Autodesk Fusion 360 part; units mm, degrees
(part 3 of 3)
sketch "Boceto17" plane through (176.3664, 0, 0) normal (1, 0, 0) x (0, 0, -1)
  line L0 (-292.5, -33.6129) -> (-292.5, -30.6129)
  line L1 (-292.5, -30.6129) -> (-354.5, -30.6129)
  line L2 (-354.5, -30.6129) -> (-354.5, -33.6129)
  line L3 (-354.5, -33.6129) -> (-292.5, -33.6129)
  line L4 (-292.5, -77.1129) -> (-292.5, 0.3871)
  line L5 (-292.5, 0.3871) -> (-357.5, 0.3871)
  line L6 (-357.5, 0.3871) -> (-357.5, -77.1129)
  line L7 (-357.5, -77.1129) -> (-292.5, -77.1129)
  line L8 (-347.5, -51.3533) -> (-347.5, -60.0136)
  line L9 (-347.5, -60.0136) -> (-352.5, -62.9003)
  line L10 (-352.5, -62.9003) -> (-352.5, -48.4666)
  line L11 (-352.5, -48.4666) -> (-347.5, -51.3533)
  line L12 (-325, -64.3437) -> (-317.5, -68.6738)
  line L13 (-317.5, -68.6738) -> (-317.5, -72.1129)
  line L14 (-317.5, -72.1129) -> (-332.5, -72.1129)
  line L15 (-332.5, -72.1129) -> (-332.5, -68.6738)
  line L16 (-332.5, -68.6738) -> (-325, -64.3437)
  line L17 (-305, -64.3437) -> (-297.5, -68.6738)
  line L18 (-297.5, -68.6738) -> (-297.5, -72.1129)
  line L19 (-297.5, -72.1129) -> (-312.5, -72.1129)
  line L20 (-312.5, -72.1129) -> (-312.5, -68.6738)
  line L21 (-312.5, -68.6738) -> (-305, -64.3437)
  line L22 (-327.5, -51.3533) -> (-327.5, -60.0136)
  line L23 (-327.5, -60.0136) -> (-335, -64.3437)
  line L24 (-335, -64.3437) -> (-342.5, -60.0136)
  line L25 (-342.5, -60.0136) -> (-342.5, -51.3533)
  line L26 (-342.5, -51.3533) -> (-335, -47.0232)
  line L27 (-335, -47.0232) -> (-327.5, -51.3533)
  line L28 (-345, -64.3437) -> (-337.5, -68.6738)
  line L29 (-337.5, -68.6738) -> (-337.5, -72.1129)
  line L30 (-337.5, -72.1129) -> (-352.5, -72.1129)
  line L31 (-352.5, -72.1129) -> (-352.5, -68.6738)
  line L32 (-352.5, -68.6738) -> (-345, -64.3437)
  line L33 (-302.5, -60.0136) -> (-302.5, -51.3533)
  line L34 (-302.5, -51.3533) -> (-297.5, -48.4666)
  line L35 (-297.5, -48.4666) -> (-297.5, -62.9003)
  line L36 (-297.5, -62.9003) -> (-302.5, -60.0136)
  line L37 (-307.5, -51.3533) -> (-307.5, -60.0136)
  line L38 (-307.5, -60.0136) -> (-315, -64.3437)
  line L39 (-315, -64.3437) -> (-322.5, -60.0136)
  line L40 (-322.5, -60.0136) -> (-322.5, -51.3533)
  line L41 (-322.5, -51.3533) -> (-315, -47.0232)
  line L42 (-315, -47.0232) -> (-307.5, -51.3533)
  line L43 (-297.5, -4.6129) -> (-297.5, -8.052)
  line L44 (-297.5, -8.052) -> (-305, -12.3822)
  line L45 (-305, -12.3822) -> (-312.5, -8.052)
  line L46 (-312.5, -8.052) -> (-312.5, -4.6129)
  line L47 (-312.5, -4.6129) -> (-297.5, -4.6129)
  line L48 (-317.5, -4.6129) -> (-317.5, -8.052)
  line L49 (-317.5, -8.052) -> (-325, -12.3822)
  line L50 (-325, -12.3822) -> (-332.5, -8.052)
  line L51 (-332.5, -8.052) -> (-332.5, -4.6129)
  line L52 (-332.5, -4.6129) -> (-317.5, -4.6129)
  line L53 (-337.5, -4.6129) -> (-337.5, -8.052)
  line L54 (-337.5, -8.052) -> (-345, -12.3822)
  line L55 (-345, -12.3822) -> (-352.5, -8.052)
  line L56 (-352.5, -8.052) -> (-352.5, -4.6129)
  line L57 (-352.5, -4.6129) -> (-337.5, -4.6129)
  line L58 (-298.6195, -27.6129) -> (-302.5, -25.3725)
  line L59 (-302.5, -25.3725) -> (-302.5, -16.7123)
  line L60 (-302.5, -16.7123) -> (-297.5, -13.8255)
  line L61 (-297.5, -13.8255) -> (-297.5, -27.6129)
  line L62 (-297.5, -27.6129) -> (-298.6195, -27.6129)
  line L63 (-351.3805, -27.6129) -> (-352.5, -27.6129)
  line L64 (-352.5, -27.6129) -> (-352.5, -13.8255)
  line L65 (-352.5, -13.8255) -> (-347.5, -16.7123)
  line L66 (-347.5, -16.7123) -> (-347.5, -25.3725)
  line L67 (-347.5, -25.3725) -> (-351.3805, -27.6129)
  line L68 (-318.6195, -27.6129) -> (-322.5, -25.3725)
  line L69 (-322.5, -25.3725) -> (-322.5, -16.7123)
  line L70 (-322.5, -16.7123) -> (-315, -12.3822)
  line L71 (-315, -12.3822) -> (-307.5, -16.7123)
  line L72 (-307.5, -16.7123) -> (-307.5, -25.3725)
  line L73 (-307.5, -25.3725) -> (-311.3805, -27.6129)
  line L74 (-311.3805, -27.6129) -> (-318.6195, -27.6129)
  line L75 (-338.6195, -27.6129) -> (-342.5, -25.3725)
  line L76 (-342.5, -25.3725) -> (-342.5, -16.7123)
  line L77 (-342.5, -16.7123) -> (-335, -12.3822)
  line L78 (-335, -12.3822) -> (-327.5, -16.7123)
  line L79 (-327.5, -16.7123) -> (-327.5, -25.3725)
  line L80 (-327.5, -25.3725) -> (-331.3805, -27.6129)
  line L81 (-331.3805, -27.6129) -> (-338.6195, -27.6129)
  line L82 (-337.5, -36.6129) -> (-337.5, -42.693)
  line L83 (-337.5, -42.693) -> (-345, -47.0232)
  line L84 (-345, -47.0232) -> (-352.5, -42.693)
  line L85 (-352.5, -42.693) -> (-352.5, -36.6129)
  line L86 (-352.5, -36.6129) -> (-337.5, -36.6129)
  line L87 (-317.5, -36.6129) -> (-317.5, -42.693)
  line L88 (-317.5, -42.693) -> (-325, -47.0232)
  line L89 (-325, -47.0232) -> (-332.5, -42.693)
  line L90 (-332.5, -42.693) -> (-332.5, -36.6129)
  line L91 (-332.5, -36.6129) -> (-317.5, -36.6129)
  line L92 (-297.5, -36.6129) -> (-297.5, -42.693)
  line L93 (-297.5, -42.693) -> (-305, -47.0232)
  line L94 (-305, -47.0232) -> (-312.5, -42.693)
  line L95 (-312.5, -42.693) -> (-312.5, -36.6129)
  line L96 (-312.5, -36.6129) -> (-297.5, -36.6129)
  line L97 (-344.5, -30.6129) -> (-302.5, -30.6129)
  line L98 (-302.5, -30.6129) -> (-302.5, -33.6129)
  line L99 (-302.5, -33.6129) -> (-344.5, -33.6129)
  line L100 (-344.5, -33.6129) -> (-344.5, -30.6129)
extrude "Extruir15" add sketch "Boceto17" along normal blind 3 contours L1 L3 L97 L98 L99 L100 bodies 7
sketch "Boceto18" plane through (-0.6336, 0, 0) normal (-1, 0, 0) x (0, 0, 1)
  line L0 (337.5, -8.052) -> (337.5, -4.6129)
  line L1 (337.5, -4.6129) -> (352.5, -4.6129)
  line L2 (352.5, -4.6129) -> (352.5, -8.052)
  line L3 (352.5, -8.052) -> (345, -12.3822)
  line L4 (345, -12.3822) -> (337.5, -8.052)
  line L5 (307.5, -25.3725) -> (307.5, -16.7123)
  line L6 (307.5, -16.7123) -> (315, -12.3822)
  line L7 (315, -12.3822) -> (322.5, -16.7123)
  line L8 (322.5, -16.7123) -> (322.5, -25.3725)
  line L9 (322.5, -25.3725) -> (315, -29.7027)
  line L10 (315, -29.7027) -> (307.5, -25.3725)
  line L11 (347.5, -60.0136) -> (347.5, -51.3533)
  line L12 (347.5, -51.3533) -> (352.5, -48.4666)
  line L13 (352.5, -48.4666) -> (352.5, -62.9003)
  line L14 (352.5, -62.9003) -> (347.5, -60.0136)
  line L15 (317.5, -68.6738) -> (325, -64.3437)
  line L16 (325, -64.3437) -> (332.5, -68.6738)
  line L17 (332.5, -68.6738) -> (332.5, -72.1129)
  line L18 (332.5, -72.1129) -> (317.5, -72.1129)
  line L19 (317.5, -72.1129) -> (317.5, -68.6738)
  line L20 (297.5, -68.6738) -> (305, -64.3437)
  line L21 (305, -64.3437) -> (312.5, -68.6738)
  line L22 (312.5, -68.6738) -> (312.5, -72.1129)
  line L23 (312.5, -72.1129) -> (297.5, -72.1129)
  line L24 (297.5, -72.1129) -> (297.5, -68.6738)
  line L25 (327.5, -60.0136) -> (327.5, -51.3533)
  line L26 (327.5, -51.3533) -> (335, -47.0232)
  line L27 (335, -47.0232) -> (342.5, -51.3533)
  line L28 (342.5, -51.3533) -> (342.5, -60.0136)
  line L29 (342.5, -60.0136) -> (335, -64.3437)
  line L30 (335, -64.3437) -> (327.5, -60.0136)
  line L31 (337.5, -42.693) -> (337.5, -34.0328)
  line L32 (337.5, -34.0328) -> (345, -29.7027)
  line L33 (345, -29.7027) -> (352.5, -34.0328)
  line L34 (352.5, -34.0328) -> (352.5, -42.693)
  line L35 (352.5, -42.693) -> (345, -47.0232)
  line L36 (345, -47.0232) -> (337.5, -42.693)
  line L37 (347.5, -25.3725) -> (347.5, -16.7123)
  line L38 (347.5, -16.7123) -> (352.5, -13.8255)
  line L39 (352.5, -13.8255) -> (352.5, -28.2593)
  line L40 (352.5, -28.2593) -> (347.5, -25.3725)
  line L41 (317.5, -8.052) -> (317.5, -4.6129)
  line L42 (317.5, -4.6129) -> (332.5, -4.6129)
  line L43 (332.5, -4.6129) -> (332.5, -8.052)
  line L44 (332.5, -8.052) -> (325, -12.3822)
  line L45 (325, -12.3822) -> (317.5, -8.052)
  line L46 (297.5, -28.2593) -> (297.5, -13.8255)
  line L47 (297.5, -13.8255) -> (302.5, -16.7123)
  line L48 (302.5, -16.7123) -> (302.5, -25.3725)
  line L49 (302.5, -25.3725) -> (297.5, -28.2593)
  line L50 (297.5, -42.693) -> (297.5, -34.0328)
  line L51 (297.5, -34.0328) -> (305, -29.7027)
  line L52 (305, -29.7027) -> (312.5, -34.0328)
  line L53 (312.5, -34.0328) -> (312.5, -42.693)
  line L54 (312.5, -42.693) -> (305, -47.0232)
  line L55 (305, -47.0232) -> (297.5, -42.693)
  line L56 (337.5, -68.6738) -> (345, -64.3437)
  line L57 (345, -64.3437) -> (352.5, -68.6738)
  line L58 (352.5, -68.6738) -> (352.5, -72.1129)
  line L59 (352.5, -72.1129) -> (337.5, -72.1129)
  line L60 (337.5, -72.1129) -> (337.5, -68.6738)
  line L61 (302.5, -51.3533) -> (302.5, -60.0136)
  line L62 (302.5, -60.0136) -> (297.5, -62.9003)
  line L63 (297.5, -62.9003) -> (297.5, -48.4666)
  line L64 (297.5, -48.4666) -> (302.5, -51.3533)
  line L65 (307.5, -60.0136) -> (307.5, -51.3533)
  line L66 (307.5, -51.3533) -> (315, -47.0232)
  line L67 (315, -47.0232) -> (322.5, -51.3533)
  line L68 (322.5, -51.3533) -> (322.5, -60.0136)
  line L69 (322.5, -60.0136) -> (315, -64.3437)
  line L70 (315, -64.3437) -> (307.5, -60.0136)
  line L71 (332.5, -42.693) -> (325, -47.0232)
  line L72 (325, -47.0232) -> (317.5, -42.693)
  line L73 (317.5, -42.693) -> (317.5, -34.0328)
  line L74 (317.5, -34.0328) -> (325, -29.7027)
  line L75 (325, -29.7027) -> (332.5, -34.0328)
  line L76 (332.5, -34.0328) -> (332.5, -42.693)
  line L77 (327.5, -25.3725) -> (327.5, -16.7123)
  line L78 (327.5, -16.7123) -> (335, -12.3822)
  line L79 (335, -12.3822) -> (342.5, -16.7123)
  line L80 (342.5, -16.7123) -> (342.5, -25.3725)
  line L81 (342.5, -25.3725) -> (335, -29.7027)
  line L82 (335, -29.7027) -> (327.5, -25.3725)
  line L83 (297.5, -8.052) -> (297.5, -4.6129)
  line L84 (297.5, -4.6129) -> (312.5, -4.6129)
  line L85 (312.5, -4.6129) -> (312.5, -8.052)
  line L86 (312.5, -8.052) -> (305, -12.3822)
  line L87 (305, -12.3822) -> (297.5, -8.052)
  line L88 (357.5, 0.3871) -> (292.5, 0.3871)
  line L89 (292.5, 0.3871) -> (292.5, -77.1129)
  line L90 (292.5, -77.1129) -> (357.5, -77.1129)
  line L91 (357.5, -77.1129) -> (357.5, 0.3871)
  line L92 (292.5, -77.1129) -> (292.5, 0.3871)
  line L93 (292.5, 0.3871) -> (357.5, 0.3871)
  line L94 (357.5, 0.3871) -> (357.5, -77.1129)
  line L95 (357.5, -77.1129) -> (292.5, -77.1129)
  line L96 (347.5, -51.3533) -> (347.5, -60.0136)
  line L97 (347.5, -60.0136) -> (352.5, -62.9003)
  line L98 (352.5, -62.9003) -> (352.5, -48.4666)
  line L99 (352.5, -48.4666) -> (347.5, -51.3533)
  line L100 (325, -64.3437) -> (317.5, -68.6738)
  line L101 (317.5, -68.6738) -> (317.5, -72.1129)
  line L102 (317.5, -72.1129) -> (332.5, -72.1129)
  line L103 (332.5, -72.1129) -> (332.5, -68.6738)
  line L104 (332.5, -68.6738) -> (325, -64.3437)
  line L105 (305, -64.3437) -> (297.5, -68.6738)
  line L106 (297.5, -68.6738) -> (297.5, -72.1129)
  line L107 (297.5, -72.1129) -> (312.5, -72.1129)
  line L108 (312.5, -72.1129) -> (312.5, -68.6738)
  line L109 (312.5, -68.6738) -> (305, -64.3437)
  line L110 (327.5, -51.3533) -> (327.5, -60.0136)
  line L111 (327.5, -60.0136) -> (335, -64.3437)
  line L112 (335, -64.3437) -> (342.5, -60.0136)
  line L113 (342.5, -60.0136) -> (342.5, -51.3533)
  line L114 (342.5, -51.3533) -> (335, -47.0232)
  line L115 (335, -47.0232) -> (327.5, -51.3533)
  line L116 (345, -64.3437) -> (337.5, -68.6738)
  line L117 (337.5, -68.6738) -> (337.5, -72.1129)
  line L118 (337.5, -72.1129) -> (352.5, -72.1129)
  line L119 (352.5, -72.1129) -> (352.5, -68.6738)
  line L120 (352.5, -68.6738) -> (345, -64.3437)
  line L121 (302.5, -60.0136) -> (302.5, -51.3533)
  line L122 (302.5, -51.3533) -> (297.5, -48.4666)
  line L123 (297.5, -48.4666) -> (297.5, -62.9003)
  line L124 (297.5, -62.9003) -> (302.5, -60.0136)
  line L125 (307.5, -51.3533) -> (307.5, -60.0136)
  line L126 (307.5, -60.0136) -> (315, -64.3437)
  line L127 (315, -64.3437) -> (322.5, -60.0136)
  line L128 (322.5, -60.0136) -> (322.5, -51.3533)
  line L129 (322.5, -51.3533) -> (315, -47.0232)
  line L130 (315, -47.0232) -> (307.5, -51.3533)
  line L131 (297.5, -4.6129) -> (297.5, -8.052)
  line L132 (297.5, -8.052) -> (305, -12.3822)
  line L133 (305, -12.3822) -> (312.5, -8.052)
  line L134 (312.5, -8.052) -> (312.5, -4.6129)
  line L135 (312.5, -4.6129) -> (297.5, -4.6129)
  line L136 (317.5, -4.6129) -> (317.5, -8.052)
  line L137 (317.5, -8.052) -> (325, -12.3822)
  line L138 (325, -12.3822) -> (332.5, -8.052)
  line L139 (332.5, -8.052) -> (332.5, -4.6129)
  line L140 (332.5, -4.6129) -> (317.5, -4.6129)
  line L141 (337.5, -4.6129) -> (337.5, -8.052)
  line L142 (337.5, -8.052) -> (345, -12.3822)
  line L143 (345, -12.3822) -> (352.5, -8.052)
  line L144 (352.5, -8.052) -> (352.5, -4.6129)
  line L145 (352.5, -4.6129) -> (337.5, -4.6129)
  line L146 (298.6195, -27.6129) -> (302.5, -25.3725)
  line L147 (302.5, -25.3725) -> (302.5, -16.7123)
  line L148 (302.5, -16.7123) -> (297.5, -13.8255)
  line L149 (297.5, -13.8255) -> (297.5, -27.6129)
  line L150 (297.5, -27.6129) -> (298.6195, -27.6129)
  line L151 (351.3805, -27.6129) -> (352.5, -27.6129)
  line L152 (352.5, -27.6129) -> (352.5, -13.8255)
  line L153 (352.5, -13.8255) -> (347.5, -16.7123)
  line L154 (347.5, -16.7123) -> (347.5, -25.3725)
  line L155 (347.5, -25.3725) -> (351.3805, -27.6129)
  line L156 (318.6195, -27.6129) -> (322.5, -25.3725)
  line L157 (322.5, -25.3725) -> (322.5, -16.7123)
  line L158 (322.5, -16.7123) -> (315, -12.3822)
  line L159 (315, -12.3822) -> (307.5, -16.7123)
  line L160 (307.5, -16.7123) -> (307.5, -25.3725)
  line L161 (307.5, -25.3725) -> (311.3805, -27.6129)
  line L162 (311.3805, -27.6129) -> (318.6195, -27.6129)
  line L163 (338.6195, -27.6129) -> (342.5, -25.3725)
  line L164 (342.5, -25.3725) -> (342.5, -16.7123)
  line L165 (342.5, -16.7123) -> (335, -12.3822)
  line L166 (335, -12.3822) -> (327.5, -16.7123)
  line L167 (327.5, -16.7123) -> (327.5, -25.3725)
  line L168 (327.5, -25.3725) -> (331.3805, -27.6129)
  line L169 (331.3805, -27.6129) -> (338.6195, -27.6129)
  line L170 (337.5, -36.6129) -> (337.5, -42.693)
  line L171 (337.5, -42.693) -> (345, -47.0232)
  line L172 (345, -47.0232) -> (352.5, -42.693)
  line L173 (352.5, -42.693) -> (352.5, -36.6129)
  line L174 (352.5, -36.6129) -> (337.5, -36.6129)
  line L175 (317.5, -36.6129) -> (317.5, -42.693)
  line L176 (317.5, -42.693) -> (325, -47.0232)
  line L177 (325, -47.0232) -> (332.5, -42.693)
  line L178 (332.5, -42.693) -> (332.5, -36.6129)
  line L179 (332.5, -36.6129) -> (317.5, -36.6129)
  line L180 (297.5, -36.6129) -> (297.5, -42.693)
  line L181 (297.5, -42.693) -> (305, -47.0232)
  line L182 (305, -47.0232) -> (312.5, -42.693)
  line L183 (312.5, -42.693) -> (312.5, -36.6129)
  line L184 (312.5, -36.6129) -> (297.5, -36.6129)
  line L185 (344.5, -30.6129) -> (302.5, -30.6129)
  line L186 (302.5, -30.6129) -> (302.5, -33.6129)
  line L187 (302.5, -33.6129) -> (344.5, -33.6129)
  line L188 (344.5, -33.6129) -> (344.5, -30.6129)
  line L189 (344.5, -33.6129) -> (302.5, -33.6129)
  line L190 (302.5, -33.6129) -> (302.5, -30.6129)
  line L191 (302.5, -30.6129) -> (344.5, -30.6129)
  line L192 (344.5, -30.6129) -> (344.5, -33.6129)
  line L193 (344.5, -33.6129) -> (344.5, -30.6129)
  line L194 (344.5, -33.6129) -> (302.5, -33.6129)
  line L195 (302.5, -33.6129) -> (302.5, -30.6129)
  line L196 (302.5, -30.6129) -> (344.5, -30.6129)
  line L197 (344.5, -30.6129) -> (344.5, -33.6129)
  line L198 (352.5, -36.6129) -> (357.5, -36.6129)
  line L199 (357.5, -36.6129) -> (292.5, -36.6129)
  line L200 (292.5, -36.6129) -> (292.5, -27.6129)
  line L201 (292.5, -27.6129) -> (357.5, -27.6129)
  line L202 (357.5, -27.6129) -> (357.5, -36.6129)
  constraint coincident L187.end L188.start
  constraint coincident L185.start L188.end
  constraint horizontal L194
  constraint vertical L195
  constraint horizontal L196
  constraint vertical L197
  constraint coincident L185.end L186.start
  constraint coincident L173.end L174.start
  constraint coincident L94 L198.end
  constraint perpendicular L94 L198
  constraint horizontal L199
  constraint vertical L200
  constraint horizontal L201
  constraint vertical L202
  constraint coincident L92 L200.end
extrude "Extruir16" add sketch "Boceto18" against normal blind 3 contours L9 L10 L162 L201 | L9 L10 L32 L33 L34 L39 L40 L46 L49 L50 L51 L52 L74 L75 L81 L82 L89 L91 L92 L94 L185 L186 L190 L191 L195 L196 L198 L199 L200 L201 L202 | L46 L49 L150 L201 | L81 L82 L169 L201 | L50 L51 L52 L53 L184 L186 L187 L189 L190 L194 L195 L199 | L52 L53 L73 L74 L187 L189 L194 L199 | L73 L74 L75 L76 L179 L187 L189 L194 L199 | L31 L32 L33 L34 L174 L185 L187 L188 L189 L191 L192 L193 L194 L196 L197 L199 | L51 L52 L185 L191 L196 | L31 L32 L75 L76 L187 L189 L194 L199 | L74 L75 L185 L191 L196 bodies 3
extrude "Extruir17" cut sketch "Boceto18" against normal blind 3 contours L51 L185 L186 L190 L191 L195 L196 | L51 L52 L185 L186 L187 L189 L190 L191 L194 L195 L196 | L52 L74 L185 L187 L189 L191 L194 L196 | L74 L75 L185 L187 L189 L191 L194 L196 | L32 L75 L185 L187 L189 L191 L194 L196 | L32 L185 L187 L188 L189 L191 L192 L193 L194 L196 L197 bodies 3
sketch "Boceto19" plane through (-0.6336, 0, 0) normal (-1, 0, 0) x (0, 0, 1)
  line L0 (344.5, -33.6129) -> (302.5, -33.6129)
  line L1 (302.5, -33.6129) -> (302.5, -30.6129)
  line L2 (302.5, -30.6129) -> (344.5, -30.6129)
  line L3 (344.5, -30.6129) -> (344.5, -33.6129)
extrude "Extruir18" add sketch "Boceto19" against normal blind 3 bodies 7
sketch "Boceto20" plane through (0, -33.6129, 0) normal (0, -1, 0) x (1, 0, 0)
  line L0 (136.8664, 296.5) -> (41.8664, 296.5)
  line L1 (41.8664, 296.5) -> (41.8664, 300.5)
  line L2 (41.8664, 300.5) -> (136.8664, 300.5)
  line L3 (136.8664, 300.5) -> (136.8664, 296.5)
  line L4 (2.3664, 292.5) -> (176.3664, 292.5)
  line L5 (176.3664, 354.5) -> (2.3664, 354.5)
  line L6 (7.3664, 349.5) -> (171.3664, 349.5)
  line L7 (171.3664, 349.5) -> (171.3664, 297.5)
  line L8 (7.3664, 297.5) -> (7.3664, 349.5)
  line L9 (41.8664, 296.5) -> (41.8664, 297.5)
  line L10 (141.8664, 305.5) -> (141.8664, 297.5)
  line L11 (171.3664, 297.5) -> (141.8664, 297.5)
  line L12 (36.8664, 297.5) -> (7.3664, 297.5)
  line L13 (36.8664, 297.5) -> (36.8664, 305.5)
  line L14 (7.3664, 323.5) -> (171.3664, 323.5) construction
  line L15 (80.7061, 323.5) -> (85.0363, 316)
  line L16 (85.0363, 316) -> (93.6965, 316)
  line L17 (93.6965, 316) -> (98.0267, 323.5)
  line L18 (98.0267, 323.5) -> (93.6965, 331)
  line L19 (93.6965, 331) -> (85.0363, 331)
  line L20 (85.0363, 331) -> (80.7061, 323.5)
  line L21 (89.3664, 323.5) -> (89.3664, 316) construction
  line L22 (89.3664, 323.5) -> (82.8712, 319.75) construction
  line L23 (169.6181, 349.5) -> (171.6388, 346)
  line L24 (171.6388, 341) -> (167.3087, 333.5)
  line L25 (167.3087, 333.5) -> (171.6388, 326)
  line L26 (171.6388, 321) -> (167.3087, 313.5)
  line L27 (167.3087, 313.5) -> (171.6388, 306)
  line L28 (171.6388, 301) -> (169.6181, 297.5)
  line L29 (153.4523, 349.5) -> (149.9882, 343.5)
  line L30 (149.9882, 343.5) -> (154.3183, 336)
  line L31 (154.3183, 336) -> (162.9786, 336)
  line L32 (167.3087, 343.5) -> (163.8446, 349.5)
  line L33 (162.9786, 336) -> (167.3087, 343.5)
  line L34 (162.9786, 331) -> (154.3183, 331)
  line L35 (154.3183, 331) -> (149.9882, 323.5)
  line L36 (149.9882, 323.5) -> (154.3183, 316)
  line L37 (154.3183, 316) -> (162.9786, 316)
  line L38 (167.3087, 323.5) -> (162.9786, 331)
  line L39 (162.9786, 316) -> (167.3087, 323.5)
  line L40 (162.9786, 311) -> (154.3183, 311)
  line L41 (154.3183, 311) -> (149.9882, 303.5)
  line L42 (149.9882, 303.5) -> (153.4523, 297.5)
  line L43 (167.3087, 303.5) -> (162.9786, 311)
  line L44 (163.8446, 297.5) -> (167.3087, 303.5)
  line L45 (134.9771, 349.5) -> (136.9978, 346)
  line L46 (136.9978, 346) -> (145.6581, 346)
  line L47 (145.6581, 346) -> (147.6788, 349.5)
  line L48 (145.6581, 341) -> (136.9978, 341)
  line L49 (136.9978, 341) -> (132.6677, 333.5)
  line L50 (132.6677, 333.5) -> (136.9978, 326)
  line L51 (136.9978, 326) -> (145.6581, 326)
  line L52 (149.9882, 333.5) -> (145.6581, 341)
  line L53 (145.6581, 326) -> (149.9882, 333.5)
  line L54 (145.6581, 321) -> (136.9978, 321)
  line L55 (136.9978, 321) -> (132.6677, 313.5)
  line L56 (132.6677, 313.5) -> (136.9978, 306)
  line L57 (136.9978, 306) -> (145.6581, 306)
  line L58 (149.9882, 313.5) -> (145.6581, 321)
  line L59 (145.6581, 306) -> (149.9882, 313.5)
  line L60 (145.6581, 301) -> (141.8664, 301)
  line L61 (136.9978, 301) -> (136.7091, 300.5)
  line L62 (147.6788, 297.5) -> (145.6581, 301)
  line L63 (118.8113, 349.5) -> (115.3472, 343.5)
  line L64 (115.3472, 343.5) -> (119.6773, 336)
  line L65 (119.6773, 336) -> (128.3375, 336)
  line L66 (132.6677, 343.5) -> (129.2036, 349.5)
  line L67 (128.3375, 336) -> (132.6677, 343.5)
  line L68 (128.3375, 331) -> (119.6773, 331)
  line L69 (119.6773, 331) -> (115.3472, 323.5)
  line L70 (115.3472, 323.5) -> (119.6773, 316)
  line L71 (119.6773, 316) -> (128.3375, 316)
  line L72 (132.6677, 323.5) -> (128.3375, 331)
  line L73 (128.3375, 316) -> (132.6677, 323.5)
  line L74 (128.3375, 311) -> (119.6773, 311)
  line L75 (119.6773, 311) -> (116.5019, 305.5)
  line L76 (131.513, 305.5) -> (128.3375, 311)
  line L77 (100.3361, 349.5) -> (102.3568, 346)
  line L78 (102.3568, 346) -> (111.017, 346)
  line L79 (111.017, 346) -> (113.0378, 349.5)
  line L80 (111.017, 341) -> (102.3568, 341)
  line L81 (102.3568, 341) -> (98.0267, 333.5)
  line L82 (98.0267, 333.5) -> (102.3568, 326)
  line L83 (102.3568, 326) -> (111.017, 326)
  line L84 (115.3472, 333.5) -> (111.017, 341)
  line L85 (111.017, 326) -> (115.3472, 333.5)
  line L86 (111.017, 321) -> (102.3568, 321)
  line L87 (102.3568, 321) -> (98.0267, 313.5)
  line L88 (98.0267, 313.5) -> (102.3568, 306)
  line L89 (102.3568, 306) -> (111.017, 306)
  line L90 (115.3472, 313.5) -> (111.017, 321)
  line L91 (111.017, 306) -> (115.3472, 313.5)
  line L92 (84.1703, 349.5) -> (80.7061, 343.5)
  line L93 (80.7061, 343.5) -> (85.0363, 336)
  line L94 (85.0363, 336) -> (93.6965, 336)
  line L95 (98.0267, 343.5) -> (94.5626, 349.5)
  line L96 (93.6965, 336) -> (98.0267, 343.5)
  line L97 (93.6965, 311) -> (85.0363, 311)
  line L98 (85.0363, 311) -> (81.8609, 305.5)
  line L99 (96.872, 305.5) -> (93.6965, 311)
  line L100 (65.695, 349.5) -> (67.7158, 346)
  line L101 (67.7158, 346) -> (76.376, 346)
  line L102 (76.376, 346) -> (78.3967, 349.5)
  line L103 (76.376, 341) -> (67.7158, 341)
  line L104 (67.7158, 341) -> (63.3856, 333.5)
  line L105 (63.3856, 333.5) -> (67.7158, 326)
  line L106 (67.7158, 326) -> (76.376, 326)
  line L107 (80.7061, 333.5) -> (76.376, 341)
  line L108 (76.376, 326) -> (80.7061, 333.5)
  line L109 (76.376, 321) -> (67.7158, 321)
  line L110 (67.7158, 321) -> (63.3856, 313.5)
  line L111 (63.3856, 313.5) -> (67.7158, 306)
  line L112 (67.7158, 306) -> (76.376, 306)
  line L113 (80.7061, 313.5) -> (76.376, 321)
  line L114 (76.376, 306) -> (80.7061, 313.5)
  line L115 (49.5292, 349.5) -> (46.0651, 343.5)
  line L116 (46.0651, 343.5) -> (50.3953, 336)
  line L117 (50.3953, 336) -> (59.0555, 336)
  line L118 (63.3856, 343.5) -> (59.9215, 349.5)
  line L119 (59.0555, 336) -> (63.3856, 343.5)
  line L120 (59.0555, 331) -> (50.3953, 331)
  line L121 (50.3953, 331) -> (46.0651, 323.5)
  line L122 (46.0651, 323.5) -> (50.3953, 316)
  line L123 (50.3953, 316) -> (59.0555, 316)
  line L124 (63.3856, 323.5) -> (59.0555, 331)
  line L125 (59.0555, 316) -> (63.3856, 323.5)
  line L126 (59.0555, 311) -> (50.3953, 311)
  line L127 (50.3953, 311) -> (47.2198, 305.5)
  line L128 (50.1066, 296.5) -> (50.3953, 296)
  line L129 (62.2309, 305.5) -> (59.0555, 311)
  line L130 (31.054, 349.5) -> (33.0748, 346)
  line L131 (33.0748, 346) -> (41.735, 346)
  line L132 (41.735, 346) -> (43.7557, 349.5)
  line L133 (41.735, 341) -> (33.0748, 341)
  line L134 (33.0748, 341) -> (28.7446, 333.5)
  line L135 (28.7446, 333.5) -> (33.0748, 326)
  line L136 (33.0748, 326) -> (41.735, 326)
  line L137 (46.0651, 333.5) -> (41.735, 341)
  line L138 (41.735, 326) -> (46.0651, 333.5)
  line L139 (41.735, 321) -> (33.0748, 321)
  line L140 (33.0748, 321) -> (28.7446, 313.5)
  line L141 (28.7446, 313.5) -> (33.0748, 306)
  line L142 (33.0748, 306) -> (41.735, 306)
  line L143 (46.0651, 313.5) -> (41.735, 321)
  line L144 (41.735, 306) -> (46.0651, 313.5)
  line L145 (36.8664, 301) -> (33.0748, 301)
  line L146 (33.0748, 301) -> (31.054, 297.5)
  line L147 (42.0237, 300.5) -> (41.735, 301)
  line L148 (14.8882, 349.5) -> (11.4241, 343.5)
  line L149 (11.4241, 343.5) -> (15.7542, 336)
  line L150 (15.7542, 336) -> (24.4145, 336)
  line L151 (28.7446, 343.5) -> (25.2805, 349.5)
  line L152 (24.4145, 336) -> (28.7446, 343.5)
  line L153 (24.4145, 331) -> (15.7542, 331)
  line L154 (15.7542, 331) -> (11.4241, 323.5)
  line L155 (11.4241, 323.5) -> (15.7542, 316)
  line L156 (15.7542, 316) -> (24.4145, 316)
  line L157 (28.7446, 323.5) -> (24.4145, 331)
  line L158 (24.4145, 316) -> (28.7446, 323.5)
  line L159 (24.4145, 311) -> (15.7542, 311)
  line L160 (15.7542, 311) -> (11.4241, 303.5)
  line L161 (11.4241, 303.5) -> (14.8882, 297.5)
  line L162 (28.7446, 303.5) -> (24.4145, 311)
  line L163 (25.2805, 297.5) -> (28.7446, 303.5)
  line L164 (7.094, 346) -> (9.1147, 349.5)
  line L165 (11.4241, 333.5) -> (7.094, 341)
  line L166 (7.094, 326) -> (11.4241, 333.5)
  line L167 (11.4241, 313.5) -> (7.094, 321)
  line L168 (7.094, 306) -> (11.4241, 313.5)
  line L169 (9.1147, 297.5) -> (7.094, 301)
  line L170 (59.0555, 296) -> (59.3442, 296.5)
  line L171 (36.8664, 305.5) -> (62.2309, 305.5)
  line L172 (81.8609, 305.5) -> (141.8664, 305.5)
  line L173 (81.8609, 305.5) -> (62.2309, 305.5)
  point P0 (89.3664, 323.5)
  dimension "d102" = 15
  constraint vertical L9
  constraint collinear L11 L12
  constraint coincident L1 L9.end
  constraint horizontal L14
  constraint coincident L7 L14.end
  constraint midpoint L14 P0
  constraint parallel L6 L19
  constraint coincident P0 L21.start
  constraint midpoint L16 L21.end
  constraint midpoint L15 L22.end
  constraint coincident L6 L23.start
  constraint coincident L6 L32.end
  constraint coincident L6 L29.start
  constraint coincident L6 L47.end
  constraint coincident L6 L45.start
  constraint coincident L6 L79.end
  constraint coincident L6 L77.start
  constraint coincident L6 L66.end
  constraint coincident L6 L63.start
  constraint coincident L6 L95.end
  constraint coincident L6 L92.start
  constraint coincident L6 L102.end
  constraint coincident L6 L100.start
  constraint coincident L6 L132.end
  constraint coincident L6 L118.end
  constraint coincident L6 L115.start
  constraint coincident L6 L130.start
  constraint coincident L6 L164.end
  constraint coincident L6 L151.end
  constraint coincident L6 L148.start
  constraint coincident L12 L169.start
  constraint coincident L12 L163.start
  constraint coincident L12 L161.end
  constraint coincident L12 L146.end
  constraint coincident L0 L170.end
  constraint coincident L0 L128.start
  constraint coincident L2 L147.start
  constraint coincident L13 L145.start
  constraint coincident L127.end L171
  constraint collinear L171 L172
  constraint coincident L172 L99.start
  constraint coincident L172 L76.start
  constraint coincident L172 L75.end
  constraint coincident L10 L60.end
  constraint coincident L2 L61.end
  constraint coincident L11 L62.start
  constraint coincident L11 L44.start
  constraint coincident L11 L42.end
  constraint coincident L11 L28.end
  constraint parallel L171 L173
  measures "d102" distance of L16 L19
extrude "Extruir19" cut sketch "Boceto20" against normal blind 40 contours L6 L148 L149 L150 L151 L152 | L6 L130 L131 L132 | L6 L115 L116 L117 L118 L119 | L6 L100 L101 L102 | L12 L159 L160 L161 L162 L163 | L6 L92 L93 L94 L95 L96 | L6 L77 L78 L79 | L6 L63 L64 L65 L66 L67 | L126 L127 L129 L171 | L6 L45 L46 L47 | L97 L98 L99 L172 | L6 L29 L30 L31 L32 L33 | L74 L75 L76 L172 | L11 L40 L41 L42 L43 L44 | L15 L16 L17 L18 L19 L20 | L34 L35 L36 L37 L38 L39 | L48 L49 L50 L51 L52 L53 | L54 L55 L56 L57 L58 L59 | L68 L69 L70 L71 L72 L73 | L80 L81 L82 L83 L84 L85 | L86 L87 L88 L89 L90 L91 | L103 L104 L105 L106 L107 L108 | L109 L110 L111 L112 L113 L114 | L120 L121 L122 L123 L124 L125 | L133 L134 L135 L136 L137 L138 | L139 L140 L141 L142 L143 L144 | L153 L154 L155 L156 L157 L158 bodies 7
move_face "CarasDesfase1" offset -0.15 2 faces at (136.8664, -117.6129, 314.1667) (41.8664, -117.6129, 314.1667) on bodies 6
move_face "CarasDesfase2" offset -0.15 4 faces at (178.3664, -33.6129, 316.5) (178.3664, -32.6129, 302.5) (178.3664, -30.6129, 316.5) (178.3664, -32.6129, 344.5) on bodies 2
sketch "Boceto21" plane through (0, 0, 292.5) normal (0, 0, -1) x (-1, 0, 0)
  line L0 (-42.0164, -116.6129) -> (-136.7164, -116.6129)
  line L1 (-136.7164, -116.6129) -> (-136.7164, -119.6129)
  line L2 (-136.7164, -119.6129) -> (-42.0164, -119.6129)
  line L3 (-42.0164, -119.6129) -> (-42.0164, -116.6129)
  line L4 (-89.3664, -116.6129) -> (-101.1964, -116.6129)
  line L5 (-101.1964, -116.6129) -> (-101.1964, -76.4129)
  line L6 (-101.1964, -76.4129) -> (-77.5364, -76.4129)
  line L7 (-77.5364, -76.4129) -> (-77.5364, -116.6129)
  line L8 (-77.5364, -116.6129) -> (-89.3664, -116.6129)
  dimension "d111" = 11.83
  dimension "d112" = 40.2
  dimension "d113" = 23.66
  constraint midpoint L0 L4.start
  constraint parallel L0 L4
  constraint perpendicular L0 L5
  constraint perpendicular L5 L6
  constraint coincident L0 L7.end
  constraint perpendicular L0 L7
  measures "d111" distance of L4.start L4.end
  measures "d112" distance of L4.end L5.end
  measures "d113" distance of L5.end L6.end
extrude "Extruir20" add sketch "Boceto21" against normal blind 2 contours L0 L4 L5 L6 L7 L8 bodies 6
sketch "Boceto22" plane through (0, 0, 294.5) normal (0, 0, 1) x (1, 0, 0)
  line L0 (77.5364, -76.4129) -> (77.5364, -116.6129)
  line L1 (77.5364, -116.6129) -> (101.1964, -116.6129)
  line L2 (101.1964, -116.6129) -> (101.1964, -76.4129)
  line L3 (101.1964, -76.4129) -> (77.5364, -76.4129)
  line L4 (77.5364, -76.4129) -> (82.0364, -76.4129)
  line L5 (82.0364, -76.4129) -> (82.0364, -86.4129)
  line L6 (82.0364, -86.4129) -> (77.5364, -86.4129)
  line L7 (77.5364, -86.4129) -> (77.5364, -76.4129)
  line L8 (101.1964, -76.4129) -> (96.6964, -76.4129)
  line L9 (96.6964, -76.4129) -> (96.6964, -86.4129)
  line L10 (96.6964, -86.4129) -> (101.1964, -86.4129)
  line L11 (101.1964, -86.4129) -> (101.1964, -76.4129)
  dimension "d116" = 4.5
  dimension "d117" = 10
  dimension "d118" = 4.5
  dimension "d119" = 10
  constraint horizontal L4
  constraint vertical L5
  constraint horizontal L6
  constraint vertical L7
  constraint coincident L0.start L3.end
  constraint horizontal L8
  constraint vertical L9
  constraint horizontal L10
  constraint vertical L11
  constraint coincident L2.end L3.start
  measures "d116" distance of L0.start L4.end
  measures "d117" distance of L0.start L6.end
  measures "d118" distance of L2.end L8.end
  measures "d119" distance of L2.end L10.end
extrude "Extruir21" add sketch "Boceto22" along normal blind 4.5 contours L0 L3 L4 L5 L6 L7 | L2 L3 L8 L9 L10 L11 bodies 6
sketch "Boceto23" plane through (0, -76.4129, 0) normal (0, 1, 0) x (-1, 0, 0)
  line L0 (-101.1964, 292.5) -> (-77.5364, 292.5)
  line L1 (-77.5364, 292.5) -> (-77.5364, 299)
  line L2 (-77.5364, 299) -> (-82.0364, 299)
  line L3 (-82.0364, 299) -> (-82.0364, 294.5)
  line L4 (-82.0364, 294.5) -> (-96.6964, 294.5)
  line L5 (-96.6964, 294.5) -> (-96.6964, 299)
  line L6 (-96.6964, 299) -> (-101.1964, 299)
  line L7 (-101.1964, 299) -> (-101.1964, 292.5)
  line L8 (-96.6964, 294.5) -> (-99.6964, 294.5)
  line L9 (-99.6964, 294.5) -> (-99.6964, 297.5)
  line L10 (-99.6964, 297.5) -> (-96.6964, 297.5)
  line L11 (-96.6964, 297.5) -> (-96.6964, 294.5)
  line L12 (-82.0364, 294.5) -> (-79.0364, 294.5)
  line L13 (-79.0364, 294.5) -> (-79.0364, 297.5)
  line L14 (-79.0364, 297.5) -> (-82.0364, 297.5)
  line L15 (-82.0364, 297.5) -> (-82.0364, 294.5)
  dimension "d122" = 3
  dimension "d123" = 3
  dimension "d124" = 3
  dimension "d125" = 3
  constraint horizontal L8
  constraint vertical L9
  constraint horizontal L10
  constraint vertical L11
  constraint coincident L4.end L5.start
  constraint horizontal L12
  constraint vertical L13
  constraint horizontal L14
  constraint vertical L15
  constraint coincident L3.end L4.start
  measures "d122" distance of L4.end L8.end
  measures "d123" distance of L4.end L10.end
  measures "d124" distance of L3.end L12.end
  measures "d125" distance of L3.end L14.end
extrude "Extruir22" cut sketch "Boceto23" against normal blind 18 contours L5 L8 L9 L10 L11 | L3 L12 L13 L14 L15 bodies 6
named bodies: "no usar", "no usar _"
